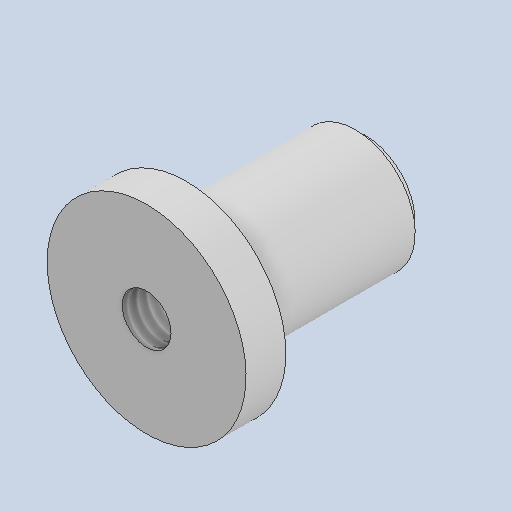
# Autodesk Inventor part: axe_taraude_m4
Saved by Autodesk Inventor 2024 (Build 280153000, 153)
## iProperties
Created: 2022-09-30
Part Number: axe_taraude_m4
Material: Générique
Document SubType Name: Modeling
Designer: ropertth
Density: 1 g/cm^3
Appearance: Par défaut
Author: ropertth
Autodesk Inventor part; units mm, degrees
ref_plane "YZ Plane" through (0, 0, 0) normal (1, 0, 0) x (0, 1, 0)
ref_plane "XZ Plane" through (0, 0, 0) normal (0, 1, 0) x (-1, 0, 0)
ref_plane "XY Plane" through (0, 0, 0) normal (0, 0, 1) x (1, 0, 0)
sketch "Esquisse1" plane through (0, 0, 0) normal (1, 0, 0) x (0, 1, 0)
  line L0 (0, 0) -> (5, 0)
  line L1 (5, 0) -> (5, -2)
  line L2 (5, -2) -> (3, -2)
  line L3 (3, -2) -> (3, -11)
  line L4 (3, -11) -> (0, -11)
  line L5 (0, -11) -> (0, 0)
  dimension "d1" = 2
  dimension "d2" = 9
  dimension "d3" = 3
  dimension "d4" = 5
  constraints: 12 end point, 5 perpendicular, 1 horizontal
  measures "d1" distance of L0.end L1.end
  measures "d2" distance of L2.end L3.end
  measures "d3" distance of L3.end L4.end
  measures "d4" distance of L0.start L0.end
revolve "Révolution1" add sketch "Esquisse1" angle 360 about axis through (0, 0, -11) along (0, 0, 1)
sketch "Esquisse2" plane through (0, 0, -11) normal (0, 0, -1) x (-1, 0, 0)
  point P0 (0, 0)
  point P1 (0, 0)
  constraints: 1 coincident
hole "Perçage1" at (0, 0, -11) direction (0, 0, 1) diameter 2.459 end through all thread size "M3x0.5" class "6H" standard "ANSI Metric M Profile"
chamfer "Chanfrein1" distance 0.5 angle 45 1 edges at (0, -3, -11)
